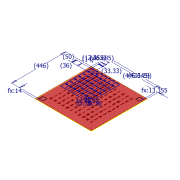
# Autodesk Inventor part: Deckblatt_schweizerdeutsch
Saved by Autodesk Inventor 2021.3 (Build 253353000, 353)
## iProperties
Part Number: Deckblatt_schweizerdeutsch
Material: Edelstahl
Document SubType Name: Modeling
Designer: fanki
Density: 8 g/cm^3
Appearance: Glatt - rot
Mass: 1626.3 g
Surface Area: 4174.16 cm^2
Volume: 203.288 cm^3
ROT_Weight: 1.626 kg
ROT_Weight_Num: 1.6263044157109727
Author: fanki
Autodesk Inventor part; units mm, degrees
(part 1 of 6)
ref_plane "YZ Plane" through (0, 0, 0) normal (1, 0, 0) x (0, 1, 0)
ref_plane "XZ Plane" through (0, 0, 0) normal (0, 1, 0) x (-1, 0, 0)
ref_plane "XY Plane" through (0, 0, 0) normal (0, 0, 1) x (1, 0, 0)
sketch "Skizze1" plane through (0, 0, 0) normal (0, 0, 1) x (1, 0, 0)
  line L0 (-210, 210) -> (210, 210) construction
  line L1 (210, 210) -> (210, -210) construction
  line L2 (210, -210) -> (-210, -210) construction
  line L3 (-210, -210) -> (-210, 210) construction
  line L4 (-230, 230) -> (230, 230)
  line L5 (230, 230) -> (230, -230)
  line L6 (230, -230) -> (-230, -230)
  line L7 (-230, -230) -> (-230, 230)
  point P0 (0, 230)
  point P1 (-230, 0)
  point P2 (-210, 0)
  point P3 (0, 210)
  point P4 (0, 0)
  point P5 (0, -210)
  point P6 (0, -230)
  dimension "d36" = 460
  dimension "d43" = 420
  constraints: 16 end point, 6 midpoint, 4 coincident, 4 parallel, 4 perpendicular, 2 horizontal, 2 horizontal alignment, 2 vertical alignment
  measures "d36" distance of L4.start L4.end
  measures "d43" distance of L0.start L0.end
extrude "Grundrahmen" add sketch "Skizze1" along normal blind 1
hole "Minuten" at (-210, 210, 0) at (210, 210, 0) at (210, -210, 0) at (-210, -210, 0) direction (0, 0, 1) diameter 4 end through all
sketch "Text" plane through (0, 0, 0) normal (0, 0, -1) x (-1, 0, 0)
  circle A0 centre (-210, -210) radius 2 projected
  circle A1 centre (210, 210) radius 2 projected
  circle A2 centre (-210, 210) radius 2 projected
  circle A3 centre (210, -210) radius 2 projected
  line L0 (230, 230) -> (-230, 230) projected
  line L1 (-230, 230) -> (-230, -230) projected
  line L2 (-230, -230) -> (230, -230) projected
  line L3 (230, -230) -> (230, 230) projected
  line L4 (183.3333, -208.5) -> (-183.3333, -208.5) construction
  line L5 (-183.3333, -208.5) -> (-183.3333, 158.1667) construction
  line L6 (-183.3333, 158.1667) -> (183.3333, 158.1667) construction
  line L7 (183.3333, 158.1667) -> (183.3333, -208.5) construction
  line L8 (-183.3333, 184.8333) -> (-150, 184.8333) construction
  line L9 (-150, 184.8333) -> (-150, 151.5) construction
  line L10 (-150, 151.5) -> (-183.3333, 151.5) construction
  line L11 (-183.3333, 151.5) -> (-183.3333, 184.8333) construction
  line L12 (-116.6667, 184.8333) -> (-83.3333, 184.8333) construction
  line L13 (-83.3333, 184.8333) -> (-83.3333, 151.5) construction
  line L14 (-83.3333, 151.5) -> (-116.6667, 151.5) construction
  line L15 (-116.6667, 151.5) -> (-116.6667, 184.8333) construction
  line L16 (-83.3333, 184.8333) -> (-50, 184.8333) construction
  line L17 (-50, 184.8333) -> (-50, 151.5) construction
  line L18 (-50, 151.5) -> (-83.3333, 151.5) construction
  line L19 (-83.3333, 151.5) -> (-83.3333, 184.8333) construction
  line L20 (-50, 184.8333) -> (-16.6667, 184.8333) construction
  line L21 (-16.6667, 184.8333) -> (-16.6667, 151.5) construction
  line L22 (-16.6667, 151.5) -> (-50, 151.5) construction
  line L23 (-50, 151.5) -> (-50, 184.8333) construction
  line L24 (-16.6667, 151.5) -> (-16.6667, 184.8333) construction
  line L25 (-16.6667, 184.8333) -> (16.6667, 184.8333) construction
  line L26 (16.6667, 184.8333) -> (16.6667, 151.5) construction
  line L27 (16.6667, 151.5) -> (-16.6667, 151.5) construction
  line L28 (16.6667, 151.5) -> (16.6667, 184.8333) construction
  line L29 (16.6667, 184.8333) -> (50, 184.8333) construction
  line L30 (50, 184.8333) -> (50, 151.5) construction
  line L31 (50, 151.5) -> (16.6667, 151.5) construction
  line L32 (50, 151.5) -> (50, 184.8333) construction
  line L33 (50, 184.8333) -> (83.3333, 184.8333) construction
  line L34 (83.3333, 184.8333) -> (83.3333, 151.5) construction
  line L35 (83.3333, 151.5) -> (50, 151.5) construction
  line L36 (83.3333, 151.5) -> (83.3333, 184.8333) construction
  line L37 (83.3333, 184.8333) -> (116.6667, 184.8333) construction
  line L38 (116.6667, 184.8333) -> (116.6667, 151.5) construction
  line L39 (116.6667, 151.5) -> (83.3333, 151.5) construction
  line L40 (116.6667, 151.5) -> (116.6667, 184.8333) construction
  line L41 (116.6667, 184.8333) -> (150, 184.8333) construction
  line L42 (150, 184.8333) -> (150, 151.5) construction
  line L43 (150, 151.5) -> (116.6667, 151.5) construction
  line L44 (150, 151.5) -> (150, 184.8333) construction
  line L45 (150, 184.8333) -> (183.3333, 184.8333) construction
  line L46 (183.3333, 184.8333) -> (183.3333, 151.5) construction
  line L47 (183.3333, 151.5) -> (150, 151.5) construction
  line L48 (-150, 148.8333) -> (-116.6667, 148.8333) construction
  line L49 (-116.6667, 148.8333) -> (-116.6667, 115.5) construction
  line L50 (-116.6667, 115.5) -> (-150, 115.5) construction
  line L51 (-150, 115.5) -> (-150, 148.8333) construction
  line L52 (-183.3333, 148.8333) -> (-150, 148.8333) construction
  line L53 (-150, 148.8333) -> (-150, 115.5) construction
  line L54 (-150, 115.5) -> (-183.3333, 115.5) construction
  line L55 (-183.3333, 115.5) -> (-183.3333, 148.8333) construction
  line L56 (230, 230) -> (-230, 230) projected
  line L57 (-230, 230) -> (-230, -230) projected
  line L58 (-116.6667, 115.5) -> (-116.6667, 148.8333) construction
  line L59 (-116.6667, 148.8333) -> (-83.3333, 148.8333) construction
  line L60 (-83.3333, 148.8333) -> (-83.3333, 115.5) construction
  line L61 (-83.3333, 115.5) -> (-116.6667, 115.5) construction
  line L62 (-83.3333, 115.5) -> (-83.3333, 148.8333) construction
  line L63 (-83.3333, 148.8333) -> (-50, 148.8333) construction
  line L64 (-50, 148.8333) -> (-50, 115.5) construction
  line L65 (-50, 115.5) -> (-83.3333, 115.5) construction
  line L66 (-50, 115.5) -> (-50, 148.8333) construction
  line L67 (-50, 148.8333) -> (-16.6667, 148.8333) construction
  line L68 (-16.6667, 148.8333) -> (-16.6667, 115.5) construction
  line L69 (-16.6667, 115.5) -> (-50, 115.5) construction
  line L70 (-16.6667, 115.5) -> (-16.6667, 148.8333) construction
  line L71 (-16.6667, 148.8333) -> (16.6667, 148.8333) construction
  line L72 (16.6667, 148.8333) -> (16.6667, 115.5) construction
  line L73 (16.6667, 115.5) -> (-16.6667, 115.5) construction
  line L74 (16.6667, 115.5) -> (16.6667, 148.8333) construction
  line L75 (16.6667, 148.8333) -> (50, 148.8333) construction
  line L76 (50, 148.8333) -> (50, 115.5) construction
  line L77 (50, 115.5) -> (16.6667, 115.5) construction
  line L78 (50, 115.5) -> (50, 148.8333) construction
  line L79 (50, 148.8333) -> (83.3333, 148.8333) construction
  line L80 (83.3333, 148.8333) -> (83.3333, 115.5) construction
  line L81 (83.3333, 115.5) -> (50, 115.5) construction
  line L82 (83.3333, 115.5) -> (83.3333, 148.8333) construction
  line L83 (83.3333, 148.8333) -> (116.6667, 148.8333) construction
  line L84 (116.6667, 148.8333) -> (116.6667, 115.5) construction
  line L85 (116.6667, 115.5) -> (83.3333, 115.5) construction
  line L86 (115.3333, 115.5) -> (115.3333, 151.5) construction
  line L87 (115.3333, 151.5) -> (151.3333, 151.5) construction
  line L88 (151.3333, 151.5) -> (151.3333, 115.5) construction
  line L89 (151.3333, 115.5) -> (115.3333, 115.5) construction
  line L90 (148.6667, 115.5) -> (148.6667, 151.5) construction
  line L91 (148.6667, 151.5) -> (184.6667, 151.5) construction
  line L92 (184.6667, 151.5) -> (184.6667, 115.5) construction
  line L93 (184.6667, 115.5) -> (148.6667, 115.5) construction
  line L94 (-183.3333, 79.5) -> (-183.3333, 112.8333) construction
  line L95 (-183.3333, 112.8333) -> (-150, 112.8333) construction
  line L96 (-150, 112.8333) -> (-150, 79.5) construction
  line L97 (-150, 79.5) -> (-183.3333, 79.5) construction
  line L98 (-150, 79.5) -> (-150, 112.8333) construction
  line L99 (-150, 112.8333) -> (-116.6667, 112.8333) construction
  line L100 (-116.6667, 112.8333) -> (-116.6667, 79.5) construction
  line L101 (-116.6667, 79.5) -> (-150, 79.5) construction
  line L102 (-116.6667, 79.5) -> (-116.6667, 112.8333) construction
  line L103 (-116.6667, 112.8333) -> (-83.3333, 112.8333) construction
  line L104 (-83.3333, 112.8333) -> (-83.3333, 79.5) construction
  line L105 (-83.3333, 79.5) -> (-116.6667, 79.5) construction
  line L106 (-83.3333, 79.5) -> (-83.3333, 112.8333) construction
  line L107 (-83.3333, 112.8333) -> (-50, 112.8333) construction
  line L108 (-50, 112.8333) -> (-50, 79.5) construction
  line L109 (-50, 79.5) -> (-83.3333, 79.5) construction
  line L110 (-50, 79.5) -> (-50, 112.8333) construction
  line L111 (-50, 112.8333) -> (-16.6667, 112.8333) construction
  line L112 (-16.6667, 112.8333) -> (-16.6667, 79.5) construction
  line L113 (-16.6667, 79.5) -> (-50, 79.5) construction
  line L114 (-16.6667, 79.5) -> (-16.6667, 112.8333) construction
  line L115 (-16.6667, 112.8333) -> (16.6667, 112.8333) construction
  line L116 (16.6667, 112.8333) -> (16.6667, 79.5) construction
  line L117 (16.6667, 79.5) -> (-16.6667, 79.5) construction
  line L118 (16.6667, 79.5) -> (16.6667, 112.8333) construction
  line L119 (16.6667, 112.8333) -> (50, 112.8333) construction
  line L120 (50, 112.8333) -> (50, 79.5) construction
  line L121 (50, 79.5) -> (16.6667, 79.5) construction
  line L122 (50, 79.5) -> (50, 112.8333) construction
  line L123 (50, 112.8333) -> (83.3333, 112.8333) construction
  line L124 (83.3333, 112.8333) -> (83.3333, 79.5) construction
  line L125 (83.3333, 79.5) -> (50, 79.5) construction
  line L126 (83.3333, 79.5) -> (83.3333, 112.8333) construction
  line L127 (83.3333, 112.8333) -> (116.6667, 112.8333) construction
  line L128 (116.6667, 112.8333) -> (116.6667, 79.5) construction
  line L129 (116.6667, 79.5) -> (83.3333, 79.5) construction
  line L130 (116.6667, 79.5) -> (116.6667, 112.8333) construction
  line L131 (116.6667, 112.8333) -> (150, 112.8333) construction
  line L132 (150, 112.8333) -> (150, 79.5) construction
  line L133 (150, 79.5) -> (116.6667, 79.5) construction
  line L134 (150, 79.5) -> (150, 112.8333) construction
  line L135 (150, 112.8333) -> (183.3333, 112.8333) construction
  line L136 (183.3333, 112.8333) -> (183.3333, 79.5) construction
  line L137 (183.3333, 79.5) -> (150, 79.5) construction
  line L138 (-183.3333, 43.5) -> (-183.3333, 76.8333) construction
  line L139 (-183.3333, 76.8333) -> (-150, 76.8333) construction
  line L140 (-150, 76.8333) -> (-150, 43.5) construction
  line L141 (-150, 43.5) -> (-183.3333, 43.5) construction
  line L142 (-150, 43.5) -> (-150, 76.8333) construction
  line L143 (-150, 76.8333) -> (-116.6667, 76.8333) construction
  line L144 (-116.6667, 76.8333) -> (-116.6667, 43.5) construction
  line L145 (-116.6667, 43.5) -> (-150, 43.5) construction
  line L146 (-116.6667, 43.5) -> (-116.6667, 76.8333) construction
  line L147 (-116.6667, 76.8333) -> (-83.3333, 76.8333) construction
  line L148 (-83.3333, 76.8333) -> (-83.3333, 43.5) construction
  line L149 (-83.3333, 43.5) -> (-116.6667, 43.5) construction
  line L150 (-83.3333, 43.5) -> (-83.3333, 76.8333) construction
  line L151 (-83.3333, 76.8333) -> (-50, 76.8333) construction
  line L152 (-50, 76.8333) -> (-50, 43.5) construction
  line L153 (-50, 43.5) -> (-83.3333, 43.5) construction
  line L154 (-50, 43.5) -> (-50, 76.8333) construction
  line L155 (-50, 76.8333) -> (-16.6667, 76.8333) construction
  line L156 (-16.6667, 76.8333) -> (-16.6667, 43.5) construction
  line L157 (-16.6667, 43.5) -> (-50, 43.5) construction
  line L158 (-16.6667, 43.5) -> (-16.6667, 76.8333) construction
  line L159 (-16.6667, 76.8333) -> (16.6667, 76.8333) construction
  line L160 (16.6667, 76.8333) -> (16.6667, 43.5) construction
  line L161 (16.6667, 43.5) -> (-16.6667, 43.5) construction
  line L162 (16.6667, 43.5) -> (16.6667, 76.8333) construction
  line L163 (16.6667, 76.8333) -> (50, 76.8333) construction
  line L164 (50, 76.8333) -> (50, 43.5) construction
  line L165 (50, 43.5) -> (16.6667, 43.5) construction
  line L166 (50, 43.5) -> (50, 76.8333) construction
  line L167 (50, 76.8333) -> (83.3333, 76.8333) construction
  line L168 (83.3333, 76.8333) -> (83.3333, 43.5) construction
  line L169 (83.3333, 43.5) -> (50, 43.5) construction
  line L170 (83.3333, 43.5) -> (83.3333, 76.8333) construction
  line L171 (83.3333, 76.8333) -> (116.6667, 76.8333) construction
  line L172 (116.6667, 76.8333) -> (116.6667, 43.5) construction
  line L173 (116.6667, 43.5) -> (83.3333, 43.5) construction
  line L174 (116.6667, 43.5) -> (116.6667, 76.8333) construction
  line L175 (116.6667, 76.8333) -> (150, 76.8333) construction
  line L176 (150, 76.8333) -> (150, 43.5) construction
  line L177 (150, 43.5) -> (116.6667, 43.5) construction
  line L178 (150, 43.5) -> (150, 76.8333) construction
  line L179 (150, 76.8333) -> (183.3333, 76.8333) construction
  line L180 (183.3333, 76.8333) -> (183.3333, 43.5) construction
  line L181 (183.3333, 43.5) -> (150, 43.5) construction
  line L182 (-183.3333, -28.5) -> (-183.3333, 4.8333) construction
  line L183 (-183.3333, 4.8333) -> (-150, 4.8333) construction
  line L184 (-150, 4.8333) -> (-150, -28.5) construction
  line L185 (-150, -28.5) -> (-183.3333, -28.5) construction
  line L186 (-150, -28.5) -> (-150, 4.8333) construction
  line L187 (-150, 4.8333) -> (-116.6667, 4.8333) construction
  line L188 (-116.6667, 4.8333) -> (-116.6667, -28.5) construction
  line L189 (-116.6667, -28.5) -> (-150, -28.5) construction
  line L190 (-116.6667, -28.5) -> (-116.6667, 4.8333) construction
  line L191 (-116.6667, 4.8333) -> (-83.3333, 4.8333) construction
  line L192 (-83.3333, 4.8333) -> (-83.3333, -28.5) construction
  line L193 (-83.3333, -28.5) -> (-116.6667, -28.5) construction
  line L194 (-83.3333, -28.5) -> (-83.3333, 4.8333) construction
  line L195 (-83.3333, 4.8333) -> (-50, 4.8333) construction
  line L196 (-50, 4.8333) -> (-50, -28.5) construction
  line L197 (-50, -28.5) -> (-83.3333, -28.5) construction
  line L198 (-50, -28.5) -> (-50, 4.8333) construction
  line L199 (-50, 4.8333) -> (-16.6667, 4.8333) construction
  line L200 (-16.6667, 4.8333) -> (-16.6667, -28.5) construction
  line L201 (-16.6667, -28.5) -> (-50, -28.5) construction
  line L202 (-16.6667, -28.5) -> (-16.6667, 4.8333) construction
  line L203 (-16.6667, 4.8333) -> (16.6667, 4.8333) construction
  line L204 (16.6667, 4.8333) -> (16.6667, -28.5) construction
  line L205 (16.6667, -28.5) -> (-16.6667, -28.5) construction
  line L206 (50, -28.5) -> (50, 4.8333) construction
  line L207 (50, 4.8333) -> (83.3333, 4.8333) construction
  line L208 (83.3333, 4.8333) -> (83.3333, -28.5) construction
  line L209 (83.3333, -28.5) -> (50, -28.5) construction
  line L210 (83.3333, -28.5) -> (83.3333, 4.8333) construction
  line L211 (83.3333, 4.8333) -> (116.6667, 4.8333) construction
  line L212 (116.6667, 4.8333) -> (116.6667, -28.5) construction
  line L213 (116.6667, -28.5) -> (83.3333, -28.5) construction
  line L214 (116.6667, -28.5) -> (116.6667, 4.8333) construction
  line L215 (116.6667, 4.8333) -> (150, 4.8333) construction
  line L216 (150, 4.8333) -> (150, -28.5) construction
  line L217 (150, -28.5) -> (116.6667, -28.5) construction
  line L218 (150, -28.5) -> (150, 4.8333) construction
  line L219 (150, 4.8333) -> (183.3333, 4.8333) construction
  line L220 (183.3333, 4.8333) -> (183.3333, -28.5) construction
  line L221 (183.3333, -28.5) -> (150, -28.5) construction
  line L222 (16.6667, -28.5) -> (16.6667, 4.8333) construction
  line L223 (16.6667, 4.8333) -> (50, 4.8333) construction
  line L224 (50, 4.8333) -> (50, -28.5) construction
  line L225 (50, -28.5) -> (16.6667, -28.5) construction
  line L226 (-183.3333, -64.5) -> (-183.3333, -31.1667) construction
  line L227 (-183.3333, -31.1667) -> (-150, -31.1667) construction
  line L228 (-150, -31.1667) -> (-150, -64.5) construction
  line L229 (-150, -64.5) -> (-183.3333, -64.5) construction
  line L230 (-150, -64.5) -> (-150, -31.1667) construction
  line L231 (-150, -31.1667) -> (-116.6667, -31.1667) construction
  line L232 (-116.6667, -31.1667) -> (-116.6667, -64.5) construction
  line L233 (-116.6667, -64.5) -> (-150, -64.5) construction
  line L234 (-116.6667, -64.5) -> (-116.6667, -31.1667) construction
  line L235 (-116.6667, -31.1667) -> (-83.3333, -31.1667) construction
  line L236 (-83.3333, -31.1667) -> (-83.3333, -64.5) construction
  line L237 (-83.3333, -64.5) -> (-116.6667, -64.5) construction
  line L238 (-83.3333, -64.5) -> (-83.3333, -31.1667) construction
  line L239 (-83.3333, -31.1667) -> (-50, -31.1667) construction
  line L240 (-50, -31.1667) -> (-50, -64.5) construction
  line L241 (-50, -64.5) -> (-83.3333, -64.5) construction
  line L242 (-50, -64.5) -> (-50, -31.1667) construction
  line L243 (-50, -31.1667) -> (-16.6667, -31.1667) construction
  line L244 (-16.6667, -31.1667) -> (-16.6667, -64.5) construction
  line L245 (-16.6667, -64.5) -> (-50, -64.5) construction
  line L246 (-16.6667, -64.5) -> (-16.6667, -31.1667) construction
  line L247 (-16.6667, -31.1667) -> (16.6667, -31.1667) construction
  line L248 (16.6667, -31.1667) -> (16.6667, -64.5) construction
  line L249 (16.6667, -64.5) -> (-16.6667, -64.5) construction
  line L250 (16.6667, -64.5) -> (16.6667, -31.1667) construction
  line L251 (16.6667, -31.1667) -> (50, -31.1667) construction
  line L252 (50, -31.1667) -> (50, -64.5) construction
  line L253 (50, -64.5) -> (16.6667, -64.5) construction
  line L254 (50, -64.5) -> (50, -31.1667) construction
  line L255 (50, -31.1667) -> (83.3333, -31.1667) construction
  line L256 (83.3333, -31.1667) -> (83.3333, -64.5) construction
  line L257 (83.3333, -64.5) -> (50, -64.5) construction
  line L258 (83.3333, -64.5) -> (83.3333, -31.1667) construction
  line L259 (83.3333, -31.1667) -> (116.6667, -31.1667) construction
  line L260 (116.6667, -31.1667) -> (116.6667, -64.5) construction
  line L261 (116.6667, -64.5) -> (83.3333, -64.5) construction
  line L262 (116.6667, -64.5) -> (116.6667, -31.1667) construction
  line L263 (116.6667, -31.1667) -> (150, -31.1667) construction
  line L264 (150, -31.1667) -> (150, -64.5) construction
  line L265 (150, -64.5) -> (116.6667, -64.5) construction
  line L266 (150, -64.5) -> (150, -31.1667) construction
  line L267 (150, -31.1667) -> (183.3333, -31.1667) construction
  line L268 (183.3333, -31.1667) -> (183.3333, -64.5) construction
  line L269 (183.3333, -64.5) -> (150, -64.5) construction
  line L270 (-183.3333, -100.5) -> (-183.3333, -67.1667) construction
  line L271 (-183.3333, -67.1667) -> (-150, -67.1667) construction
  line L272 (-150, -67.1667) -> (-150, -100.5) construction
  line L273 (-150, -100.5) -> (-183.3333, -100.5) construction
  line L274 (-16.6667, -100.5) -> (-16.6667, -67.1667) construction
  line L275 (-16.6667, -67.1667) -> (16.6667, -67.1667) construction
  line L276 (16.6667, -67.1667) -> (16.6667, -100.5) construction
  line L277 (16.6667, -100.5) -> (-16.6667, -100.5) construction
  line L278 (-50, -100.5) -> (-50, -67.1667) construction
  line L279 (-50, -67.1667) -> (-16.6667, -67.1667) construction
  line L280 (-16.6667, -67.1667) -> (-16.6667, -100.5) construction
  line L281 (-16.6667, -100.5) -> (-50, -100.5) construction
  line L282 (-83.3333, -100.5) -> (-83.3333, -67.1667) construction
  line L283 (-83.3333, -67.1667) -> (-50, -67.1667) construction
  line L284 (-50, -67.1667) -> (-50, -100.5) construction
  line L285 (-50, -100.5) -> (-83.3333, -100.5) construction
  line L286 (-116.6667, -100.5) -> (-116.6667, -67.1667) construction
  line L287 (-116.6667, -67.1667) -> (-83.3333, -67.1667) construction
  line L288 (-83.3333, -67.1667) -> (-83.3333, -100.5) construction
  line L289 (-83.3333, -100.5) -> (-116.6667, -100.5) construction
  line L290 (-150, -100.5) -> (-150, -67.1667) construction
  line L291 (-150, -67.1667) -> (-116.6667, -67.1667) construction
  line L292 (-116.6667, -67.1667) -> (-116.6667, -100.5) construction
  line L293 (-116.6667, -100.5) -> (-150, -100.5) construction
  line L294 (16.6667, -100.5) -> (16.6667, -67.1667) construction
  line L295 (16.6667, -67.1667) -> (50, -67.1667) construction
  line L296 (50, -67.1667) -> (50, -100.5) construction
  line L297 (50, -100.5) -> (16.6667, -100.5) construction
  line L298 (50, -100.5) -> (50, -67.1667) construction
  line L299 (50, -67.1667) -> (83.3333, -67.1667) construction
  line L300 (83.3333, -67.1667) -> (83.3333, -100.5) construction
  line L301 (83.3333, -100.5) -> (50, -100.5) construction
  line L302 (83.3333, -100.5) -> (83.3333, -67.1667) construction
  line L303 (83.3333, -67.1667) -> (116.6667, -67.1667) construction
  line L304 (116.6667, -67.1667) -> (116.6667, -100.5) construction
  line L305 (116.6667, -100.5) -> (83.3333, -100.5) construction
  line L306 (116.6667, -100.5) -> (116.6667, -67.1667) construction
  line L307 (116.6667, -67.1667) -> (150, -67.1667) construction
  line L308 (150, -67.1667) -> (150, -100.5) construction
  line L309 (150, -100.5) -> (116.6667, -100.5) construction
  line L310 (150, -100.5) -> (150, -67.1667) construction
  line L311 (150, -67.1667) -> (183.3333, -67.1667) construction
  line L312 (183.3333, -67.1667) -> (183.3333, -100.5) construction
  line L313 (183.3333, -100.5) -> (150, -100.5) construction
  line L314 (-183.3333, -136.5) -> (-183.3333, -103.1667) construction
  line L315 (-183.3333, -103.1667) -> (-150, -103.1667) construction
  line L316 (-150, -103.1667) -> (-150, -136.5) construction
  line L317 (-150, -136.5) -> (-183.3333, -136.5) construction
  line L318 (-150, -136.5) -> (-150, -103.1667) construction
  line L319 (-150, -103.1667) -> (-116.6667, -103.1667) construction
  line L320 (-116.6667, -103.1667) -> (-116.6667, -136.5) construction
  line L321 (-116.6667, -136.5) -> (-150, -136.5) construction
  line L322 (-116.6667, -136.5) -> (-116.6667, -103.1667) construction
  line L323 (-116.6667, -103.1667) -> (-83.3333, -103.1667) construction
  line L324 (-83.3333, -103.1667) -> (-83.3333, -136.5) construction
  line L325 (-83.3333, -136.5) -> (-116.6667, -136.5) construction
  line L326 (-50, -136.5) -> (-50, -103.1667) construction
  line L327 (-50, -103.1667) -> (-16.6667, -103.1667) construction
  line L328 (-16.6667, -103.1667) -> (-16.6667, -136.5) construction
  line L329 (-16.6667, -136.5) -> (-50, -136.5) construction
  line L330 (-83.3333, -136.5) -> (-83.3333, -103.1667) construction
  line L331 (-83.3333, -103.1667) -> (-50, -103.1667) construction
  line L332 (-50, -103.1667) -> (-50, -136.5) construction
  line L333 (-50, -136.5) -> (-83.3333, -136.5) construction
  line L334 (-16.6667, -136.5) -> (-16.6667, -103.1667) construction
  line L335 (-16.6667, -103.1667) -> (16.6667, -103.1667) construction
  line L336 (16.6667, -103.1667) -> (16.6667, -136.5) construction
  line L337 (16.6667, -136.5) -> (-16.6667, -136.5) construction
  line L338 (16.6667, -136.5) -> (16.6667, -103.1667) construction
  line L339 (16.6667, -103.1667) -> (50, -103.1667) construction
  line L340 (50, -103.1667) -> (50, -136.5) construction
  line L341 (50, -136.5) -> (16.6667, -136.5) construction
  line L342 (50, -136.5) -> (50, -103.1667) construction
  line L343 (50, -103.1667) -> (83.3333, -103.1667) construction
  line L344 (83.3333, -103.1667) -> (83.3333, -136.5) construction
  line L345 (83.3333, -136.5) -> (50, -136.5) construction
  line L346 (83.3333, -136.5) -> (83.3333, -103.1667) construction
  line L347 (83.3333, -103.1667) -> (116.6667, -103.1667) construction
  line L348 (116.6667, -103.1667) -> (116.6667, -136.5) construction
  line L349 (116.6667, -136.5) -> (83.3333, -136.5) construction
  line L350 (116.6667, -136.5) -> (116.6667, -103.1667) construction
  line L351 (116.6667, -103.1667) -> (150, -103.1667) construction
  line L352 (150, -103.1667) -> (150, -136.5) construction
  line L353 (150, -136.5) -> (116.6667, -136.5) construction
  line L354 (150, -136.5) -> (150, -103.1667) construction
  line L355 (150, -103.1667) -> (183.3333, -103.1667) construction
  line L356 (183.3333, -103.1667) -> (183.3333, -136.5) construction
  line L357 (183.3333, -136.5) -> (150, -136.5) construction
  line L358 (-183.3333, -172.5) -> (-183.3333, -139.1667) construction
  line L359 (-183.3333, -139.1667) -> (-150, -139.1667) construction
  line L360 (-150, -139.1667) -> (-150, -172.5) construction
  line L361 (-150, -172.5) -> (-183.3333, -172.5) construction
  line L362 (-150, -172.5) -> (-150, -139.1667) construction
  line L363 (-150, -139.1667) -> (-116.6667, -139.1667) construction
  line L364 (-116.6667, -139.1667) -> (-116.6667, -172.5) construction
  line L365 (-116.6667, -172.5) -> (-150, -172.5) construction
  line L366 (-116.6667, -172.5) -> (-116.6667, -139.1667) construction
  line L367 (-116.6667, -139.1667) -> (-83.3333, -139.1667) construction
  line L368 (-83.3333, -139.1667) -> (-83.3333, -172.5) construction
  line L369 (-83.3333, -172.5) -> (-116.6667, -172.5) construction
  line L370 (-83.3333, -172.5) -> (-83.3333, -139.1667) construction
  line L371 (-83.3333, -139.1667) -> (-50, -139.1667) construction
  line L372 (-50, -139.1667) -> (-50, -172.5) construction
  line L373 (-50, -172.5) -> (-83.3333, -172.5) construction
  line L374 (-50, -172.5) -> (-50, -139.1667) construction
  line L375 (-50, -139.1667) -> (-16.6667, -139.1667) construction
  line L376 (-16.6667, -139.1667) -> (-16.6667, -172.5) construction
  line L377 (-16.6667, -172.5) -> (-50, -172.5) construction
  line L378 (-16.6667, -172.5) -> (-16.6667, -139.1667) construction
  line L379 (-16.6667, -139.1667) -> (16.6667, -139.1667) construction
  line L380 (16.6667, -139.1667) -> (16.6667, -172.5) construction
  line L381 (16.6667, -172.5) -> (-16.6667, -172.5) construction
  line L382 (50, -172.5) -> (50, -139.1667) construction
  line L383 (50, -139.1667) -> (83.3333, -139.1667) construction
  line L384 (83.3333, -139.1667) -> (83.3333, -172.5) construction
  line L385 (83.3333, -172.5) -> (50, -172.5) construction
  line L386 (150, -172.5) -> (150, -139.1667) construction
  line L387 (150, -139.1667) -> (183.3333, -139.1667) construction
  line L388 (183.3333, -139.1667) -> (183.3333, -172.5) construction
  line L389 (183.3333, -172.5) -> (150, -172.5) construction
  line L390 (116.6667, -172.5) -> (116.6667, -139.1667) construction
  line L391 (116.6667, -139.1667) -> (150, -139.1667) construction
  line L392 (150, -139.1667) -> (150, -172.5) construction
  line L393 (150, -172.5) -> (116.6667, -172.5) construction
  line L394 (83.3333, -172.5) -> (83.3333, -139.1667) construction
  line L395 (83.3333, -139.1667) -> (116.6667, -139.1667) construction
  line L396 (116.6667, -139.1667) -> (116.6667, -172.5) construction
  line L397 (116.6667, -172.5) -> (83.3333, -172.5) construction
  line L398 (16.6667, -172.5) -> (16.6667, -139.1667) construction
  line L399 (16.6667, -139.1667) -> (50, -139.1667) construction
  line L400 (50, -139.1667) -> (50, -172.5) construction
  line L401 (50, -172.5) -> (16.6667, -172.5) construction
  line L402 (-150, 184.8333) -> (-116.6667, 184.8333) construction
  line L403 (-116.6667, 184.8333) -> (-116.6667, 151.5) construction
  line L404 (-116.6667, 151.5) -> (-150, 151.5) construction
  line L405 (-150, 151.5) -> (-150, 184.8333) construction
  line L406 (-16.6667, 7.5) -> (-16.6667, 40.8333) construction
  line L407 (-16.6667, 40.8333) -> (16.6667, 40.8333) construction
  line L408 (16.6667, 40.8333) -> (16.6667, 7.5) construction
  line L409 (16.6667, 7.5) -> (-16.6667, 7.5) construction
  line L410 (-50, 7.5) -> (-50, 40.8333) construction
  line L411 (-50, 40.8333) -> (-16.6667, 40.8333) construction
  line L412 (-16.6667, 40.8333) -> (-16.6667, 7.5) construction
  line L413 (-16.6667, 7.5) -> (-50, 7.5) construction
  line L414 (-83.3333, 7.5) -> (-83.3333, 40.8333) construction
  line L415 (-83.3333, 40.8333) -> (-50, 40.8333) construction
  line L416 (-50, 40.8333) -> (-50, 7.5) construction
  line L417 (-50, 7.5) -> (-83.3333, 7.5) construction
  line L418 (-116.6667, 7.5) -> (-116.6667, 40.8333) construction
  line L419 (-116.6667, 40.8333) -> (-83.3333, 40.8333) construction
  line L420 (-83.3333, 40.8333) -> (-83.3333, 7.5) construction
  line L421 (-83.3333, 7.5) -> (-116.6667, 7.5) construction
  line L422 (-150, 7.5) -> (-150, 40.8333) construction
  line L423 (-150, 40.8333) -> (-116.6667, 40.8333) construction
  line L424 (-116.6667, 40.8333) -> (-116.6667, 7.5) construction
  line L425 (-116.6667, 7.5) -> (-150, 7.5) construction
  line L426 (-183.3333, 7.5) -> (-183.3333, 40.8333) construction
  line L427 (-183.3333, 40.8333) -> (-150, 40.8333) construction
  line L428 (-150, 40.8333) -> (-150, 7.5) construction
  line L429 (-150, 7.5) -> (-183.3333, 7.5) construction
  line L430 (16.6667, 7.5) -> (16.6667, 40.8333) construction
  line L431 (16.6667, 40.8333) -> (50, 40.8333) construction
  line L432 (50, 40.8333) -> (50, 7.5) construction
  line L433 (50, 7.5) -> (16.6667, 7.5) construction
  line L434 (50, 7.5) -> (50, 40.8333) construction
  line L435 (50, 40.8333) -> (83.3333, 40.8333) construction
  line L436 (83.3333, 40.8333) -> (83.3333, 7.5) construction
  line L437 (83.3333, 7.5) -> (50, 7.5) construction
  line L438 (83.3333, 7.5) -> (83.3333, 40.8333) construction
  line L439 (83.3333, 40.8333) -> (116.6667, 40.8333) construction
  line L440 (116.6667, 40.8333) -> (116.6667, 7.5) construction
  line L441 (116.6667, 7.5) -> (83.3333, 7.5) construction
  line L442 (116.6667, 7.5) -> (116.6667, 40.8333) construction
  line L443 (116.6667, 40.8333) -> (150, 40.8333) construction
  line L444 (150, 40.8333) -> (150, 7.5) construction
  line L445 (150, 7.5) -> (116.6667, 7.5) construction
  line L446 (150, 7.5) -> (150, 40.8333) construction
  line L447 (150, 40.8333) -> (183.3333, 40.8333) construction
  line L448 (183.3333, 40.8333) -> (183.3333, 7.5) construction
  line L449 (183.3333, 7.5) -> (150, 7.5) construction
  spline S0 degree 2 poles (-169.8448, 171.5518) (-169.8448, 171.9557) (-169.2829, 172.5) (-168.8966, 172.5) knots 0 0 0 1 2 2 2
  line L450 (-168.8966, 172.5) -> (-162.8213, 172.5)
  spline S1 degree 2 poles (-162.8213, 172.5) (-162.4351, 172.5) (-161.8732, 171.9557) (-161.8732, 171.5518) knots 0 0 0 1 2 2 2
  spline S2 degree 2 poles (-161.8732, 171.5518) (-161.8732, 171.1656) (-162.4351, 170.6037) (-162.8213, 170.6037) knots 0 0 0 1 2 2 2
  line L451 (-162.8213, 170.6037) -> (-167.9309, 170.6037)
  line L452 (-167.9309, 170.6037) -> (-167.9309, 162.9657)
  line L453 (-167.9309, 162.9657) -> (-163.8046, 162.9657)
  spline S3 degree 2 poles (-163.8046, 162.9657) (-163.4008, 162.9657) (-162.8389, 162.4038) (-162.8389, 162) knots 0 0 0 1 2 2 2
  spline S4 degree 2 poles (-162.8389, 162) (-162.8389, 161.6137) (-163.4008, 161.0518) (-163.8046, 161.0518) knots 0 0 0 1 2 2 2
  line L454 (-163.8046, 161.0518) -> (-167.9309, 161.0518)
  line L455 (-167.9309, 161.0518) -> (-167.9309, 153.4139)
  line L456 (-167.9309, 153.4139) -> (-162.8213, 153.4139)
  spline S5 degree 2 poles (-162.8213, 153.4139) (-162.4351, 153.4139) (-161.8732, 152.852) (-161.8732, 152.4482) knots 0 0 0 1 2 2 2
  spline S6 degree 2 poles (-161.8732, 152.4482) (-161.8732, 152.0794) (-162.4351, 151.5) (-162.8213, 151.5) knots 0 0 0 1 2 2 2
  line L457 (-162.8213, 151.5) -> (-168.8966, 151.5)
  spline S7 degree 2 poles (-168.8966, 151.5) (-169.2829, 151.5) (-169.8448, 152.0619) (-169.8448, 152.4482) knots 0 0 0 1 2 2 2
  line L458 (-169.8448, 152.4482) -> (-169.8448, 171.5518)
  spline S8 degree 2 poles (-96.5146, 171.9908) (-96.4444, 172.1137) (-96.3215, 172.2366) knots 0 0 0 1 1 1
  spline S9 degree 2 poles (-96.3215, 172.2366) (-96.0406, 172.5) (-95.6543, 172.5) knots 0 0 0 1 1 1
  spline S10 degree 2 poles (-95.6543, 172.5) (-95.2504, 172.5) (-94.7237, 171.9732) (-94.7237, 171.5694) knots 0 0 0 1 2 2 2
  spline S11 degree 2 poles (-94.7237, 171.5694) (-94.7237, 171.2709) (-94.8641, 171.0251) knots 0 0 0 1 1 1
  line L459 (-94.8641, 171.0251) -> (-98.9377, 161.842)
  line L460 (-98.9377, 161.842) -> (-94.8641, 152.9925)
  spline S12 degree 2 poles (-94.8641, 152.9925) (-94.7237, 152.7467) (-94.7237, 152.4306) knots 0 0 0 1 1 1
  spline S13 degree 2 poles (-94.7237, 152.4306) (-94.7237, 152.0443) (-95.2504, 151.5) (-95.6543, 151.5) knots 0 0 0 1 2 2 2
  spline S14 degree 2 poles (-95.6543, 151.5) (-96.0406, 151.5) (-96.3215, 151.7634) knots 0 0 0 1 1 1
  spline S15 degree 2 poles (-96.3215, 151.7634) (-96.4444, 151.9038) (-96.5146, 152.0268) knots 0 0 0 1 1 1
  line L461 (-96.5146, 152.0268) -> (-100.8165, 161.3503)
  spline S16 degree 2 poles (-100.8165, 161.3503) (-100.9569, 161.5786) (-100.9569, 161.842) knots 0 0 0 1 1 1
  spline S17 degree 2 poles (-100.9569, 161.842) (-100.9569, 162.1229) (-100.8165, 162.3336) knots 0 0 0 1 1 1
  line L462 (-100.8165, 162.3336) -> (-96.5146, 171.9908)
  spline S18 degree 2 poles (-104.135, 171.5518) (-104.135, 171.9557) (-103.5732, 172.5) (-103.1869, 172.5) knots 0 0 0 1 2 2 2
  spline S19 degree 2 poles (-103.1869, 172.5) (-102.783, 172.5) (-102.2212, 171.9557) (-102.2212, 171.5518) knots 0 0 0 1 2 2 2
  line L463 (-102.2212, 171.5518) -> (-102.2212, 152.4482)
  spline S20 degree 2 poles (-102.2212, 152.4482) (-102.2212, 152.0619) (-102.783, 151.5) (-103.1869, 151.5) knots 0 0 0 1 2 2 2
  spline S21 degree 2 poles (-103.1869, 151.5) (-103.5732, 151.5) (-104.135, 152.0619) (-104.135, 152.4482) knots 0 0 0 1 2 2 2
  line L464 (-104.135, 152.4482) -> (-104.135, 171.5518)
  spline S22 degree 2 poles (-67.6236, 171.5518) (-67.6236, 171.9557) (-67.0617, 172.5) (-66.6754, 172.5) knots 0 0 0 1 2 2 2
  spline S23 degree 2 poles (-66.6754, 172.5) (-66.2716, 172.5) (-65.7097, 171.9557) (-65.7097, 171.5518) knots 0 0 0 1 2 2 2
  line L465 (-65.7097, 171.5518) -> (-65.7097, 152.4482)
  spline S24 degree 2 poles (-65.7097, 152.4482) (-65.7097, 152.0619) (-66.2716, 151.5) (-66.6754, 151.5) knots 0 0 0 1 2 2 2
  spline S25 degree 2 poles (-66.6754, 151.5) (-67.0617, 151.5) (-67.6236, 152.0619) (-67.6236, 152.4482) knots 0 0 0 1 2 2 2
  line L466 (-67.6236, 152.4482) -> (-67.6236, 171.5518)
  spline S26 degree 2 poles (-36.8802, 152.9749) (-37.1787, 153.3261) (-37.1787, 153.7299) knots 0 0 0 1 1 1
  spline S27 degree 2 poles (-37.1787, 153.7299) (-37.1435, 154.1338) (-36.8626, 154.3972) knots 0 0 0 1 1 1
  spline S28 degree 2 poles (-36.8626, 154.3972) (-36.5992, 154.643) (-36.1778, 154.643) knots 0 0 0 1 1 1
  spline S29 degree 2 poles (-36.1778, 154.643) (-35.7915, 154.6079) (-35.4579, 154.2742) knots 0 0 0 1 1 1
  spline S30 degree 2 poles (-35.4579, 154.2742) (-34.7556, 153.4841) (-33.7021, 153.4314) knots 0 0 0 1 1 1
  line L467 (-33.7021, 153.4314) -> (-33.5792, 153.4314)
  spline S31 degree 2 poles (-33.5792, 153.4314) (-32.5959, 153.4314) (-31.876, 154.0987) knots 0 0 0 1 1 1
  spline S32 degree 2 poles (-31.876, 154.0987) (-31.0858, 154.801) (-31.0332, 155.837) knots 0 0 0 1 1 1
  line L468 (-31.0332, 155.837) -> (-31.0332, 156.0477)
  spline S33 degree 2 poles (-31.0332, 156.0477) (-31.0332, 158.6814) (-34.2288, 162.2107) knots 0 0 0 1 1 1
  spline S34 degree 2 poles (-34.2288, 162.2107) (-37.4069, 165.7224) (-37.4069, 168.6722) knots 0 0 0 1 1 1
  line L469 (-37.4069, 168.6722) -> (-37.4069, 168.9356)
  spline S35 degree 2 poles (-37.4069, 168.9356) (-37.3016, 170.7968) (-35.932, 172.0259) knots 0 0 0 1 1 1
  spline S36 degree 2 poles (-35.932, 172.0259) (-34.6502, 173.1672) (-32.9822, 173.1672) knots 0 0 0 1 1 1
  line L470 (-32.9822, 173.1672) -> (-32.7188, 173.1672)
  spline S37 degree 2 poles (-32.7188, 173.1672) (-30.8576, 173.0619) (-29.646, 171.6923) knots 0 0 0 1 1 1
  spline S38 degree 2 poles (-29.646, 171.6923) (-29.33, 171.3411) (-29.33, 170.9548) knots 0 0 0 1 1 1
  spline S39 degree 2 poles (-29.33, 170.9548) (-29.3651, 170.551) (-29.6636, 170.2876) knots 0 0 0 1 1 1
  spline S40 degree 2 poles (-29.6636, 170.2876) (-29.927, 170.0418) (-30.2957, 170.0418) knots 0 0 0 1 1 1
  spline S41 degree 2 poles (-30.2957, 170.0418) (-30.7347, 170.0594) (-31.0332, 170.4105) knots 0 0 0 1 1 1
  spline S42 degree 2 poles (-31.0332, 170.4105) (-31.7706, 171.1831) (-32.8241, 171.2358) knots 0 0 0 1 1 1
  line L471 (-32.8241, 171.2358) -> (-32.9997, 171.2358)
  spline S43 degree 2 poles (-32.9997, 171.2358) (-33.9303, 171.2358) (-34.6502, 170.6037) knots 0 0 0 1 1 1
  spline S44 degree 2 poles (-34.6502, 170.6037) (-35.4404, 169.8838) (-35.493, 168.8303) knots 0 0 0 1 1 1
  line L472 (-35.493, 168.8303) -> (-35.493, 168.6898)
  spline S45 degree 2 poles (-35.493, 168.6898) (-35.493, 166.4774) (-32.2623, 162.9306) knots 0 0 0 1 1 1
  spline S46 degree 2 poles (-32.2623, 162.9306) (-29.1017, 159.4189) (-29.1017, 156.1003) knots 0 0 0 1 1 1
  spline S47 degree 2 poles (-29.1017, 156.1003) (-29.1017, 155.9247) (-29.1193, 155.7492) knots 0 0 0 1 1 1
  spline S48 degree 2 poles (-29.1193, 155.7492) (-29.2246, 153.888) (-30.5942, 152.6413) knots 0 0 0 1 1 1
  spline S49 degree 2 poles (-30.5942, 152.6413) (-31.876, 151.5) (-33.5616, 151.5) knots 0 0 0 1 1 1
  line L473 (-33.5616, 151.5) -> (-33.8074, 151.5)
  spline S50 degree 2 poles (-33.8074, 151.5) (-35.6511, 151.6054) (-36.8802, 152.9749) knots 0 0 0 1 1 1
  spline S51 degree 2 poles (2.8094, 154.2216) (3.0727, 154.4849) (3.4766, 154.4849) knots 0 0 0 1 1 1
  spline S52 degree 2 poles (3.4766, 154.4849) (3.8629, 154.4849) (4.4247, 153.9406) (4.4247, 153.5368) knots 0 0 0 1 2 2 2
  spline S53 degree 2 poles (4.4247, 153.5368) (4.4247, 153.1505) (4.1614, 152.8696) knots 0 0 0 1 1 1
  spline S54 degree 2 poles (4.1614, 152.8696) (2.8094, 151.5) (0.9657, 151.5) knots 0 0 0 1 1 1
  spline S55 degree 2 poles (0.9657, 151.5) (-0.8955, 151.5) (-3.4941, 154.1162) (-3.4941, 155.9599) knots 0 0 0 1 2 2 2
  line L474 (-3.4941, 155.9599) -> (-3.4941, 168.7249)
  spline S56 degree 2 poles (-3.4941, 168.7249) (-3.4941, 170.5686) (-0.8955, 173.1848) (0.9657, 173.1848) knots 0 0 0 1 2 2 2
  spline S57 degree 2 poles (0.9657, 173.1848) (2.8094, 173.1848) (4.1614, 171.8152) knots 0 0 0 1 1 1
  spline S58 degree 2 poles (4.1614, 171.8152) (4.4247, 171.5167) (4.4247, 171.148) knots 0 0 0 1 1 1
  spline S59 degree 2 poles (4.4247, 171.148) (4.4247, 170.7441) (3.8629, 170.1823) (3.4766, 170.1823) knots 0 0 0 1 2 2 2
  spline S60 degree 2 poles (3.4766, 170.1823) (3.0727, 170.1823) (2.8094, 170.4632) knots 0 0 0 1 1 1
  spline S61 degree 2 poles (2.8094, 170.4632) (2.0017, 171.2533) (0.9657, 171.2533) knots 0 0 0 1 1 1
  spline S62 degree 2 poles (0.9657, 171.2533) (-0.1054, 171.2533) (-1.5803, 169.7609) (-1.5803, 168.7074) knots 0 0 0 1 2 2 2
  line L475 (-1.5803, 168.7074) -> (-1.5803, 155.9774)
  spline S63 degree 2 poles (-1.5803, 155.9774) (-1.5803, 154.9239) (-0.1054, 153.4314) (0.9657, 153.4314) knots 0 0 0 1 2 2 2
  spline S64 degree 2 poles (0.9657, 153.4314) (2.0017, 153.4314) (2.8094, 154.2216) knots 0 0 0 1 1 1
  spline S65 degree 2 poles (28.5574, 171.5518) (28.5574, 171.9557) (29.1193, 172.5) (29.5056, 172.5) knots 0 0 0 1 2 2 2
  spline S66 degree 2 poles (29.5056, 172.5) (29.9094, 172.5) (30.4713, 171.9557) (30.4713, 171.5518) knots 0 0 0 1 2 2 2
  line L476 (30.4713, 171.5518) -> (30.4713, 162.9657)
  line L477 (30.4713, 162.9657) -> (36.1778, 162.9657)
  line L478 (36.1778, 162.9657) -> (36.1778, 171.5518)
  spline S67 degree 2 poles (36.1778, 171.5518) (36.1778, 171.9557) (36.7397, 172.5) (37.1435, 172.5) knots 0 0 0 1 2 2 2
  spline S68 degree 2 poles (37.1435, 172.5) (37.5298, 172.5) (38.0917, 171.9557) (38.0917, 171.5518) knots 0 0 0 1 2 2 2
  line L479 (38.0917, 171.5518) -> (38.0917, 152.4482)
  spline S69 degree 2 poles (38.0917, 152.4482) (38.0917, 152.0619) (37.5298, 151.5) (37.1435, 151.5) knots 0 0 0 1 2 2 2
  spline S70 degree 2 poles (37.1435, 151.5) (36.7397, 151.5) (36.1778, 152.0619) (36.1778, 152.4482) knots 0 0 0 1 2 2 2
  line L480 (36.1778, 152.4482) -> (36.1778, 161.0518)
  line L481 (36.1778, 161.0518) -> (30.4713, 161.0518)
  line L482 (30.4713, 161.0518) -> (30.4713, 152.4482)
  spline S71 degree 2 poles (30.4713, 152.4482) (30.4713, 152.0619) (29.9094, 151.5) (29.5056, 151.5) knots 0 0 0 1 2 2 2
  spline S72 degree 2 poles (29.5056, 151.5) (29.1193, 151.5) (28.5574, 152.0619) (28.5574, 152.4482) knots 0 0 0 1 2 2 2
  line L483 (28.5574, 152.4482) -> (28.5574, 171.5518)
  spline S73 degree 2 poles (66.6754, 157.8211) (67.0617, 157.8211) (67.6236, 157.2592) (67.6236, 156.8554) knots 0 0 0 1 2 2 2
  spline S74 degree 2 poles (67.6236, 156.8554) (67.6236, 156.4691) (67.0617, 155.9072) (66.6754, 155.9072) knots 0 0 0 1 2 2 2
  line L484 (66.6754, 155.9072) -> (63.4974, 155.9072)
  line L485 (63.4974, 155.9072) -> (62.5316, 152.2901)
  spline S75 degree 2 poles (62.5316, 152.2901) (62.4438, 151.9916) (62.2507, 151.7809) knots 0 0 0 1 1 1
  spline S76 degree 2 poles (62.2507, 151.7809) (61.9698, 151.5) (61.5835, 151.5) knots 0 0 0 1 1 1
  spline S77 degree 2 poles (61.5835, 151.5) (61.1796, 151.5) (60.6178, 152.0619) (60.6178, 152.4482) knots 0 0 0 1 2 2 2
  spline S78 degree 2 poles (60.6178, 152.4482) (60.6178, 152.5711) (60.6353, 152.6589) knots 0 0 0 1 1 1
  line L486 (60.6353, 152.6589) -> (65.7273, 171.6572)
  spline S79 degree 2 poles (65.7273, 171.6572) (65.7975, 171.9732) (66.0082, 172.2015) knots 0 0 0 1 1 1
  spline S80 degree 2 poles (66.0082, 172.2015) (66.2892, 172.5) (66.6754, 172.5) knots 0 0 0 1 1 1
  spline S81 degree 2 poles (66.6754, 172.5) (67.0617, 172.5) (67.3602, 172.2015) knots 0 0 0 1 1 1
  spline S82 degree 2 poles (67.3602, 172.2015) (67.5358, 171.9732) (67.606, 171.6572) knots 0 0 0 1 1 1
  line L487 (67.606, 171.6572) -> (72.698, 152.6589)
  spline S83 degree 2 poles (72.698, 152.6589) (72.7156, 152.5711) (72.7156, 152.4482) knots 0 0 0 1 1 1
  spline S84 degree 2 poles (72.7156, 152.4482) (72.7156, 152.0619) (72.1537, 151.5) (71.7674, 151.5) knots 0 0 0 1 2 2 2
  spline S85 degree 2 poles (71.7674, 151.5) (71.3636, 151.5) (71.1002, 151.7809) knots 0 0 0 1 1 1
  spline S86 degree 2 poles (71.1002, 151.7809) (70.8895, 151.9916) (70.8017, 152.2901) knots 0 0 0 1 1 1
  line L488 (70.8017, 152.2901) -> (66.6754, 167.7943)
  line L489 (66.6754, 167.7943) -> (64.0065, 157.8211)
  line L490 (64.0065, 157.8211) -> (66.6754, 157.8211)
  spline S87 degree 2 poles (103.1781, 162.9657) (103.5819, 162.9657) (104.1438, 162.4038) (104.1438, 162) knots 0 0 0 1 2 2 2
  spline S88 degree 2 poles (104.1438, 162) (104.1438, 161.6137) (103.5819, 161.0518) (103.1781, 161.0518) knots 0 0 0 1 2 2 2
  line L491 (103.1781, 161.0518) -> (99.0518, 161.0518)
  line L492 (99.0518, 161.0518) -> (99.0518, 152.4482)
  spline S89 degree 2 poles (99.0518, 152.4482) (99.0518, 152.0619) (98.49, 151.5) (98.0861, 151.5) knots 0 0 0 1 2 2 2
  spline S90 degree 2 poles (98.0861, 151.5) (97.6998, 151.5) (97.138, 152.0619) (97.138, 152.4482) knots 0 0 0 1 2 2 2
  line L493 (97.138, 152.4482) -> (97.138, 171.5518)
  spline S91 degree 2 poles (97.138, 171.5518) (97.138, 171.9557) (97.6998, 172.5) (98.0861, 172.5) knots 0 0 0 1 2 2 2
  line L494 (98.0861, 172.5) -> (104.1614, 172.5)
  spline S92 degree 2 poles (104.1614, 172.5) (104.5477, 172.5) (105.1095, 171.9557) (105.1095, 171.5518) knots 0 0 0 1 2 2 2
  spline S93 degree 2 poles (105.1095, 171.5518) (105.1095, 171.1656) (104.5477, 170.6037) (104.1614, 170.6037) knots 0 0 0 1 2 2 2
  line L495 (104.1614, 170.6037) -> (99.0518, 170.6037)
  line L496 (99.0518, 170.6037) -> (99.0518, 162.9657)
  line L497 (99.0518, 162.9657) -> (103.1781, 162.9657)
  spline S94 degree 2 poles (128.8822, 171.8503) (128.8822, 172.2542) (129.4441, 172.8161) (129.8304, 172.8161) knots 0 0 0 1 2 2 2
  spline S95 degree 2 poles (129.8304, 172.8161) (130.2343, 172.8161) (130.7961, 172.2542) (130.7961, 171.8503) knots 0 0 0 1 2 2 2
  line L498 (130.7961, 171.8503) -> (130.7961, 155.9599)
  spline S96 degree 2 poles (130.7961, 155.9599) (130.7961, 154.9064) (132.2886, 153.4139) (133.3421, 153.4139) knots 0 0 0 1 2 2 2
  spline S97 degree 2 poles (133.3421, 153.4139) (134.3956, 153.4139) (135.8881, 154.9064) (135.8881, 155.9599) knots 0 0 0 1 2 2 2
  line L499 (135.8881, 155.9599) -> (135.8881, 171.8503)
  spline S98 degree 2 poles (135.8881, 171.8503) (135.8881, 172.2542) (136.4324, 172.8161) (136.8363, 172.8161) knots 0 0 0 1 2 2 2
  spline S99 degree 2 poles (136.8363, 172.8161) (137.2401, 172.8161) (137.802, 172.2542) (137.802, 171.8503) knots 0 0 0 1 2 2 2
  line L500 (137.802, 171.8503) -> (137.802, 155.9599)
  spline S100 degree 2 poles (137.802, 155.9599) (137.802, 154.1162) (135.1858, 151.5) (133.3421, 151.5) knots 0 0 0 1 2 2 2
  spline S101 degree 2 poles (133.3421, 151.5) (131.4985, 151.5) (128.8822, 154.1162) (128.8822, 155.9599) knots 0 0 0 1 2 2 2
  line L501 (128.8822, 155.9599) -> (128.8822, 171.8503)
  spline S102 degree 2 poles (135.6598, 177.9256) (136.1866, 177.9256) (136.9416, 177.1706) (136.9416, 176.6438) knots 0 0 0 1 2 2 2
  spline S103 degree 2 poles (136.9416, 176.6438) (136.9416, 176.1171) (136.1866, 175.3796) (135.6598, 175.3796) knots 0 0 0 1 2 2 2
  spline S104 degree 2 poles (135.6598, 175.3796) (135.1331, 175.3796) (134.3956, 176.1171) (134.3956, 176.6438) knots 0 0 0 1 2 2 2
  spline S105 degree 2 poles (134.3956, 176.6438) (134.3956, 177.1706) (135.1331, 177.9256) (135.6598, 177.9256) knots 0 0 0 1 2 2 2
  spline S106 degree 2 poles (131.0244, 177.9256) (131.5511, 177.9256) (132.3062, 177.1706) (132.3062, 176.6438) knots 0 0 0 1 2 2 2
  spline S107 degree 2 poles (132.3062, 176.6438) (132.3062, 176.1171) (131.5511, 175.3796) (131.0244, 175.3796) knots 0 0 0 1 2 2 2
  spline S108 degree 2 poles (131.0244, 175.3796) (130.4976, 175.3796) (129.7602, 176.1171) (129.7602, 176.6438) knots 0 0 0 1 2 2 2
  spline S109 degree 2 poles (129.7602, 176.6438) (129.7602, 177.1706) (130.4976, 177.9256) (131.0244, 177.9256) knots 0 0 0 1 2 2 2
  spline S110 degree 2 poles (169.8448, 162.9657) (170.2486, 162.9657) (170.8105, 162.4038) (170.8105, 162) knots 0 0 0 1 2 2 2
  spline S111 degree 2 poles (170.8105, 162) (170.8105, 161.6137) (170.2486, 161.0518) (169.8448, 161.0518) knots 0 0 0 1 2 2 2
  line L502 (169.8448, 161.0518) -> (165.7185, 161.0518)
  line L503 (165.7185, 161.0518) -> (165.7185, 152.4482)
  spline S112 degree 2 poles (165.7185, 152.4482) (165.7185, 152.0619) (165.1566, 151.5) (164.7528, 151.5) knots 0 0 0 1 2 2 2
  spline S113 degree 2 poles (164.7528, 151.5) (164.3665, 151.5) (163.8046, 152.0619) (163.8046, 152.4482) knots 0 0 0 1 2 2 2
  line L504 (163.8046, 152.4482) -> (163.8046, 171.5518)
  spline S114 degree 2 poles (163.8046, 171.5518) (163.8046, 171.9557) (164.3665, 172.5) (164.7528, 172.5) knots 0 0 0 1 2 2 2
  line L505 (164.7528, 172.5) -> (170.828, 172.5)
  spline S115 degree 2 poles (170.828, 172.5) (171.2143, 172.5) (171.7762, 171.9557) (171.7762, 171.5518) knots 0 0 0 1 2 2 2
  spline S116 degree 2 poles (171.7762, 171.5518) (171.7762, 171.1656) (171.2143, 170.6037) (170.828, 170.6037) knots 0 0 0 1 2 2 2
  line L506 (170.828, 170.6037) -> (165.7185, 170.6037)
  line L507 (165.7185, 170.6037) -> (165.7185, 162.9657)
  line L508 (165.7185, 162.9657) -> (169.8448, 162.9657)
  spline S117 degree 2 poles (-172.698, 135.3411) (-172.7156, 135.4465) (-172.7156, 135.5518) knots 0 0 0 1 1 1
  spline S118 degree 2 poles (-172.7156, 135.5518) (-172.7156, 135.9557) (-172.1537, 136.5) (-171.7499, 136.5) knots 0 0 0 1 2 2 2
  spline S119 degree 2 poles (-171.7499, 136.5) (-171.3636, 136.5) (-171.0826, 136.2366) knots 0 0 0 1 1 1
  spline S120 degree 2 poles (-171.0826, 136.2366) (-170.8719, 136.0084) (-170.8017, 135.7099) knots 0 0 0 1 1 1
  line L509 (-170.8017, 135.7099) -> (-166.6579, 120.1881)
  line L510 (-166.6579, 120.1881) -> (-162.5316, 135.7099)
  spline S121 degree 2 poles (-162.5316, 135.7099) (-162.4614, 136.0084) (-162.2331, 136.2366) knots 0 0 0 1 1 1
  spline S122 degree 2 poles (-162.2331, 136.2366) (-161.9698, 136.5) (-161.5659, 136.5) knots 0 0 0 1 1 1
  spline S123 degree 2 poles (-161.5659, 136.5) (-161.1796, 136.5) (-160.6178, 135.9557) (-160.6178, 135.5518) knots 0 0 0 1 2 2 2
  spline S124 degree 2 poles (-160.6178, 135.5518) (-160.6178, 135.4465) (-160.6353, 135.3411) knots 0 0 0 1 1 1
  line L511 (-160.6353, 135.3411) -> (-165.7273, 116.3253)
  spline S125 degree 2 poles (-165.7273, 116.3253) (-165.7975, 116.0268) (-165.9731, 115.7809) knots 0 0 0 1 1 1
  spline S126 degree 2 poles (-165.9731, 115.7809) (-166.2716, 115.5) (-166.6579, 115.5) knots 0 0 0 1 1 1
  spline S127 degree 2 poles (-166.6579, 115.5) (-167.0442, 115.5) (-167.3251, 115.7809) knots 0 0 0 1 1 1
  spline S128 degree 2 poles (-167.3251, 115.7809) (-167.5358, 116.0268) (-167.606, 116.3253) knots 0 0 0 1 1 1
  line L512 (-167.606, 116.3253) -> (-172.698, 135.3411)
  spline S129 degree 2 poles (-134.2903, 135.5518) (-134.2903, 135.9557) (-133.7284, 136.5) (-133.3421, 136.5) knots 0 0 0 1 2 2 2
  spline S130 degree 2 poles (-133.3421, 136.5) (-132.9383, 136.5) (-132.3764, 135.9557) (-132.3764, 135.5518) knots 0 0 0 1 2 2 2
  line L513 (-132.3764, 135.5518) -> (-132.3764, 116.4482)
  spline S131 degree 2 poles (-132.3764, 116.4482) (-132.3764, 116.0619) (-132.9383, 115.5) (-133.3421, 115.5) knots 0 0 0 1 2 2 2
  spline S132 degree 2 poles (-133.3421, 115.5) (-133.7284, 115.5) (-134.2903, 116.0619) (-134.2903, 116.4482) knots 0 0 0 1 2 2 2
  line L514 (-134.2903, 116.4482) -> (-134.2903, 135.5518)
  spline S133 degree 2 poles (-103.1781, 135.5518) (-103.1781, 135.9557) (-102.6162, 136.5) (-102.2299, 136.5) knots 0 0 0 1 2 2 2
  line L515 (-102.2299, 136.5) -> (-96.1547, 136.5)
  spline S134 degree 2 poles (-96.1547, 136.5) (-95.7684, 136.5) (-95.2065, 135.9557) (-95.2065, 135.5518) knots 0 0 0 1 2 2 2
  spline S135 degree 2 poles (-95.2065, 135.5518) (-95.2065, 135.1656) (-95.7684, 134.6037) (-96.1547, 134.6037) knots 0 0 0 1 2 2 2
  line L516 (-96.1547, 134.6037) -> (-101.2642, 134.6037)